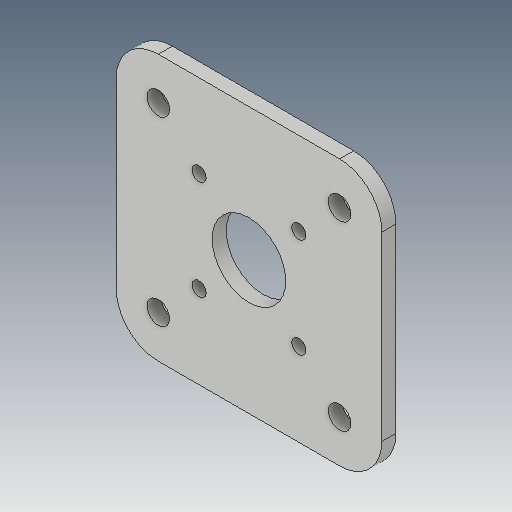
# Autodesk Inventor part: 車輪ハブ1
Saved by Autodesk Inventor 2020.3 (Build 243373000, 373)
## iProperties
Part Number: 車輪ハブ1
Material: 一般
Document SubType Name: Modeling
Designer: highs
Density: 1 g/cm^3
Appearance: 既定
Stock Number: 自作or外注　カーボン化検討
Author: highs
Autodesk Inventor part; units mm, degrees
ref_plane "YZ Plane" through (0, 0, 0) normal (1, 0, 0) x (0, 1, 0)
ref_plane "XZ Plane" through (0, 0, 0) normal (0, 1, 0) x (-1, 0, 0)
ref_plane "XY Plane" through (0, 0, 0) normal (0, 0, 1) x (1, 0, 0)
sketch "スケッチ1" plane through (0, 0, 0) normal (0, 0, 1) x (1, 0, 0)
  line L0 (-47.1734, 47.1734) -> (47.1734, 47.1734)
  line L1 (47.1734, 47.1734) -> (47.1734, -47.1734)
  line L2 (47.1734, -47.1734) -> (-47.1734, -47.1734)
  line L3 (-47.1734, -47.1734) -> (-47.1734, 47.1734)
  line L4 (-47.1734, 47.1734) -> (47.1734, -47.1734) construction
  line L5 (47.1734, 47.1734) -> (-47.1734, -47.1734) construction
  circle A0 centre (32.1734, 32.1734) radius 4
  circle A1 centre (-32.1734, 32.1734) radius 4
  circle A2 centre (-32.1734, -32.1734) radius 4
  circle A3 centre (32.1734, -32.1734) radius 4
  circle A4 centre (0, 0) radius 45.5 construction
  circle A5 centre (0, 0) radius 13.05
  circle A6 centre (0, 0) radius 25 construction
  circle A7 centre (17.6777, 17.6777) radius 2.5
  circle A8 centre (-17.6777, 17.6777) radius 2.5
  circle A9 centre (-17.6777, -17.6777) radius 2.5
  circle A10 centre (17.6777, -17.6777) radius 2.5
  line L6 (-7.8, -7.8) -> (7.8, 7.8) construction
  line L7 (7.8, -7.8) -> (-7.8, 7.8) construction
  line L8 (-17.6777, -17.6777) -> (-17.6777, 17.6777) construction
  line L9 (-17.6777, 17.6777) -> (17.6777, 17.6777) construction
  line L10 (17.6777, -17.6777) -> (-17.6777, -17.6777) construction
  line L11 (17.6777, -17.6777) -> (17.6777, 17.6777) construction
  dimension "d4" = 91
  dimension "d2" = 360
  dimension "d5" = 26.1
  dimension "d7" = 8
  dimension "d8" = 5
  dimension "d12" = 360
  dimension "d26" = 15
  dimension "d27" = 50
  constraints: 24 end point, 10 centre point, 4 midpoint, 4 point on line, 3 coincident, 3 perpendicular, 2 parallel, 2 point on circle, 1 horizontal, 1 vertical, 21 other
  measures "d5" diameter of A5
  measures "d7" diameter of A0
  measures "d8" diameter of A7
  measures "d26" distance from line of L3 A1.centre
  measures "d27" diameter of A6
extrude "押し出し2" add sketch "スケッチ1" along normal blind 5
fillet "フィレット4" radius 15 4 edges at (47.1734, -47.1734, 2.5) (47.1734, 47.1734, 2.5) (-47.1734, -47.1734, 2.5) (-47.1734, 47.1734, 2.5)
